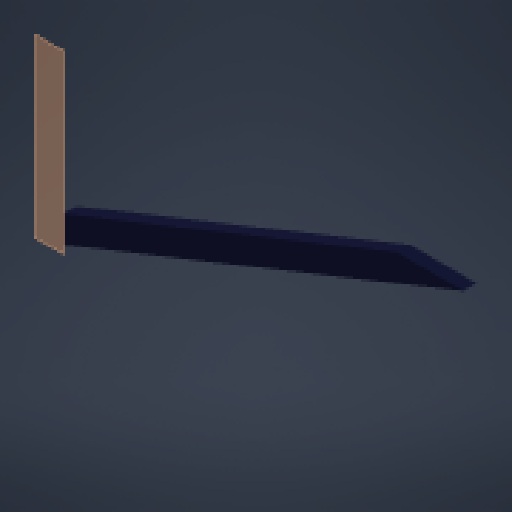
# Autodesk Inventor part: Upper side diagonal
Saved by Autodesk Inventor 2027 (Build 310192000, 192)
## iProperties
Created: 2026-05-29
Part Number: Upper side diagonal
Material: Generic
Document SubType Name: Modeling
Designer: lucas
Density: 1 g/cm^3
Appearance: Default
Author: lucas
Autodesk Inventor part; units mm, degrees
ref_plane "YZ Plane" through (0, 0, 0) normal (1, 0, 0) x (0, 1, 0)
ref_plane "XZ Plane" through (0, 0, 0) normal (0, 1, 0) x (-1, 0, 0)
ref_plane "XY Plane" through (0, 0, 0) normal (0, 0, 1) x (1, 0, 0)
ref_plane "Work Plane1" through (0, 0, 0) normal (0, 0, 1) x (1, 0, 0)
ref_plane "Work Plane2" through (0, 0, 0) normal (0, 0, 1) x (1, 0, 0)
sketch "Sketch1" plane through (0, 0, 0) normal (0, 0, 1) x (1, 0, 0)
  line L0 (50.8, 304.8) -> (-50.8, 304.8) projected
  line L1 (-50.8, 304.8) -> (-50.8, -245.3386) projected
  line L2 (-50.8, -245.3386) -> (50.8, -304.8) projected
  line L3 (50.8, -304.8) -> (50.8, 304.8) projected
  line L4 (-1041.4, 304.8) -> (1524, 304.8) projected
  line L5 (1524, 304.8) -> (1524, 406.4) projected
  line L6 (1524, 406.4) -> (-1041.4, 406.4) projected
  line L7 (-1041.4, 406.4) -> (-1041.4, 304.8) projected
  line L8 (1574.8, 304.8) -> (1574.8, 406.4) projected
  line L9 (1574.8, 406.4) -> (1524, 406.4) projected
  line L10 (1524, 304.8) -> (1524, 406.4) projected
  line L11 (1574.8, 304.8) -> (1524, 304.8) projected
  line L12 (1574.8, 304.8) -> (50.8, -304.8)
  line L13 (50.8, -203.2) -> (50.8, -304.8)
  line L14 (50.8, -203.2) -> (1320.8, 304.8)
  line L15 (1320.8, 304.8) -> (1574.8, 304.8)
  point P0 (0, 0)
  dimension "d0" = 101.6
  constraints: 8 end point, 3 point on line, 1 collinear, 1 parallel, 1 perpendicular
  measures "d0" distance of L2.end L13.start
extrude "Extrusion1" add sketch "Sketch1" against normal blind 50.8 contours L14 L4 L11 L12 L3
body "Solid1"
